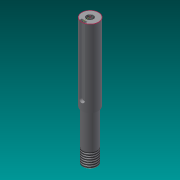
# Autodesk Inventor part: 正しい
Saved by Autodesk Inventor 2015 (Build 190159000, 159)
## iProperties
Created: 2016-02-22
Part Number: 正しい
Material: 一般
Document SubType Name: Modeling
Designer: buzztaka
Density: 1 g/cm^3
Appearance: 既定
Author: buzztaka
Autodesk Inventor part; units mm, degrees
ref_plane "YZ Plane" through (0, 0, 0) normal (1, 0, 0) x (0, 1, 0)
ref_plane "XZ Plane" through (0, 0, 0) normal (0, 1, 0) x (-1, 0, 0)
sketch "スケッチ1" plane through (0, 0, 0) normal (0, 0, 1) x (1, 0, 0)
  circle A0 centre (0, 0) radius 5
  dimension "d0" = 10
  constraints: 1 centre point, 1 coincident
  measures "d0" diameter of A0
extrude "押し出し1" add sketch "スケッチ1" along normal blind 35
thread "ねじ1" size "M10x1.5" class "6g" standard "ANSI Metric M Profile" length 10
sketch "スケッチ2" plane through (0, 0, 35) normal (0, 0, 1) x (1, 0, 0)
  circle A0 centre (0, 0) radius 6
  dimension "d5" = 12
  constraints: 1 centre point, 1 coincident
  measures "d5" diameter of A0
extrude "押し出し2" add sketch "スケッチ2" along normal blind 55
sketch "スケッチ6" plane through (0, 0, 90) normal (0, 0, 1) x (1, 0, 0)
  line L0 (0, 0) -> (0, -6) construction
  circle A0 centre (0, 0) radius 6 projected
  constraints: 2 end point, 1 vertical alignment, 1 other
ref_plane "作業平面5" through (0, -6, 90) normal (0, -1, 0) x (1, 0, 0)
sketch "スケッチ8" plane through (0, -6, 90) normal (0, -1, 0) x (1, 0, 0)
  line L0 (6, 0) -> (-6, 0) projected
  line L1 (-2, 0) -> (2, 0)
  line L2 (-2, 0) -> (2, 0)
  line L3 (2, 0) -> (2, -48)
  line L4 (-2, -48) -> (-2, 0)
  arc A0 (-2, -48) -> (2, -48) centre (0, -48) ccw
  point P0 (0, -90)
  point P1 (0, 0)
  dimension "d11" = 2
  dimension "d17" = 48
  dimension "d29" = 2
  constraints: 8 end point, 2 horizontal, 2 point on circle, 1 centre point, 1 coincident, 1 midpoint, 1 parallel, 1 perpendicular, 1 point on line
  measures "d11" distance of point (0, 0) L1.start
  measures "d17" distance of point (0, 0) point (0, -48)
  measures "d29" distance from line of L3 point (0, 0)
extrude "押し出し3" cut sketch "スケッチ8" against normal blind 2.157
sketch "スケッチ9" plane through (0, 0, 90) normal (0, 0, 1) x (1, 0, 0)
  point P0 (0, 0)
  point P1 (0, 0)
  constraints: 1 coincident
hole "穴1" at (0, 0, 90) direction (0, 0, -1) diameter 5 depth 8 tip angle 118
thread "ねじ2" size "Rc 2 1/2" standard "ISO Taper Internal" full length
thread "ねじ3" size "M5x0.8" class "6H" standard "ANSI Metric M Profile" full length
